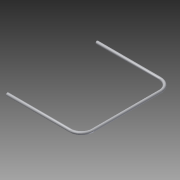
# Autodesk Inventor part: Aluminum Tube Bent 0.500 OD 0.436 ID
Saved by Autodesk Inventor 2014 (Build 180170000, 170)
## iProperties
Created: 2014-01-06
Part Number: Aluminum Tube Bent 0.500 OD 0.436 ID
Material: Aluminum 6061
Document SubType Name: Modeling
Designer: Andrew Toennies
Mass: 84.9768 g
Surface Area: 706.099 cm^2
Volume: 31.3568 cm^3
Density: 2.71 g/cm^3
Appearance: Aluminum - Flat
Author: Andrew Toennies
Autodesk Inventor part; units mm, degrees
ref_plane "YZ Plane" through (0, 0, 0) normal (1, 0, 0) x (0, 1, 0)
ref_plane "XZ Plane" through (0, 0, 0) normal (0, 1, 0) x (-1, 0, 0)
ref_plane "XY Plane" through (0, 0, 0) normal (0, 0, 1) x (1, 0, 0)
sketch "Sketch1" plane through (0, 0, 0) normal (0, 0, 1) x (1, 0, 0)
  circle A0 centre (0, 0) radius 6.35
  circle A1 centre (0, 0) radius 5.461
  dimension "d0" = 12.7
  dimension "d1" = 0.889
  constraints: 2 centre point, 1 coincident
  measures "d0" diameter of A0
  measures "d1" radial gap between concentric circles of A0 A1
sketch "Sketch2" plane through (0, 0, 0) normal (0, 1, 0) x (-1, 0, 0)
  line L0 (0, 0) -> (0, 158.75)
  arc A0 (50.8, 209.55) -> (0, 158.75) centre (50.8, 158.75) ccw
  line L1 (50.8, 158.75) -> (0, 158.75) construction
  line L2 (50.8, 209.55) -> (336.55, 209.55)
  line L3 (50.8, 158.75) -> (50.8, 209.55) construction
  line L4 (336.55, 209.55) -> (336.55, -165.107) construction
  dimension "d2" = 158.75
  dimension "d3" = 50.8
  dimension "d4" = 336.55
  constraints: 10 end point, 2 point on circle, 2 vertical, 1 centre point, 1 horizontal, 1 parallel, 1 perpendicular
  measures "d2" distance of L0.start L0.end
  measures "d3" distance of L1.start L0.end
  measures "d4" distance from line of L0 L2.end
sweep "Sweep1" add profiles "Sketch1" path "Sketch2"
mirror "Mirror1" about plane through (0, 0, 0) normal (0, 0, -1) of "Sweep1"
body "Solid1"
